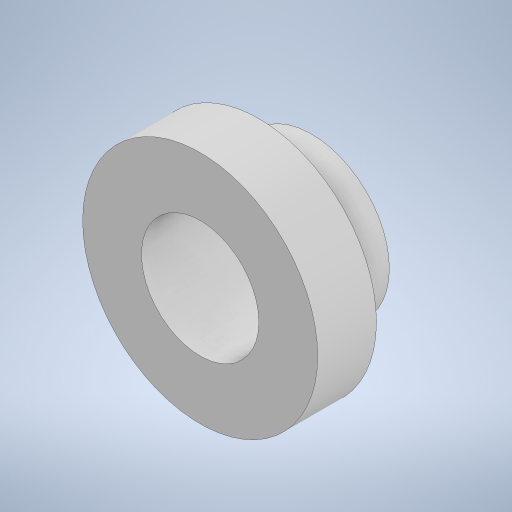
# Autodesk Inventor part: CAD_A_inner
Saved by Autodesk Inventor 2023 (Build 270158000, 158)
## iProperties
Created: 2023-05-08
Part Number: CAD_A_inner
Material: Generic
Document SubType Name: Modeling
Designer: steff
Density: 1 g/cm^3
Appearance: Default
Author: steff
## iProperties of the stored document CAD_A_inner_3DPrint.ipt
Created: 2023-05-08
Part Number: CAD_A_inner_3DPrint
Material: Generic
Document SubType Name: Modeling
Designer: steff
Density: 1 g/cm^3
Appearance: Default
Author: steff
Autodesk Inventor part; units mm, degrees
ref_plane "YZ Plane" through (0, 0, 0) normal (1, 0, 0) x (0, 1, 0)
ref_plane "XZ Plane" through (0, 0, 0) normal (0, 1, 0) x (-1, 0, 0)
ref_plane "XY Plane" through (0, 0, 0) normal (0, 0, 1) x (1, 0, 0)
sketch "Sketch1" plane through (0, 0, 0) normal (0, 0, 1) x (1, 0, 0)
  circle A0 centre (0, 0) radius 4.995
  circle A1 centre (0, 0) radius 6.6
  dimension "d0" = 9.99
  dimension "d1" = 13.2
  constraints: 2 centre point, 2 coincident
  measures "d0" diameter of A0
  measures "d1" diameter of A1
extrude "Extrusion1" add sketch "Sketch1" along normal blind 9.5
sketch "Sketch2" plane through (0, 0, 9.5) normal (0, 0, 1) x (1, 0, 0)
  circle A0 centre (0, 0) radius 6.55
  circle A1 centre (0, 0) radius 6.6 projected
  circle A2 centre (0, 0) radius 10
  dimension "d4" = 20
  constraints: 2 centre point, 2 coincident
  measures "d4" diameter of A2
extrude "Extrusion2" add sketch "Sketch2" against normal blind 5 contours A2
body "Solid1"
